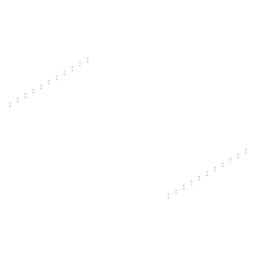
Shelf Support drillings for entire panel (Autodesk Fusion 360 design; units mm, degrees)
Autodesk Fusion 360 part; units mm, degrees
sketch "Control" plane through (0, 0, 0) normal (0, 0, 1) x (1, 0, 0)
  line L0 (378.5, -280) -> (-378.5, -280)
  line L1 (-378.5, -280) -> (-378.5, 280)
  line L2 (-378.5, 280) -> (378.5, 280)
  line L3 (378.5, 280) -> (378.5, -280)
  line L4 (378.5, -280) -> (-378.5, 280) construction
  line L5 (-378.5, -280) -> (378.5, 280) construction
  point P0 (0, 160)
  dimension "d7" = 560
  dimension "d8" = 757
  dimension "d9" = 378.5
  dimension "d100" = 120
  constraint horizontal L0
  constraint perpendicular L0 L1
  constraint parallel L0 L2
  constraint parallel L1 L3
  constraint coincident L4 origin
  constraint coincident L5 origin
  measures "d7" distance of L0.end L1.end
  measures "d8" distance of L1 L3
  measures "d9" distance of L1 P0
  measures "d100" vertical distance of L1.end P0
ref_plane "WorkPlane1" through (0, 160, 0) normal (0, 1, 0) x (0, 0, 1)
ref_plane "WorkPlane2" through (0, 0, 0) normal (1, 0, 0) x (0, 1, 0)
sketch "Sketch5" plane through (0, 0, 0) normal (0, 0, 1) x (1, 0, 0)
  line L0 (346.5, 160) -> (-346.5, 160) construction
  line L1 (-378.5, 280) -> (378.5, 280) construction
  line L2 (378.5, 280) -> (378.5, -280) construction
  line L3 (-378.5, -280) -> (-378.5, 280) construction
  circle A0 centre (-346.5, 160) radius 2.5
  circle A1 centre (346.5, 160) radius 2.5
  dimension "d116" = 120
  dimension "d117" = 32
  dimension "d118" = 32
  dimension "d119" = 5
  dimension "d120" = 5
  constraint horizontal L0
  constraint coincident L0.end A0.centre
  constraint coincident L0.start A1.centre
  measures "d116" distance of L0 L1
  measures "d117" distance of L0.end L3
  measures "d118" distance of L0.start L2
  measures "d119" diameter of A0
  measures "d120" diameter of A1
extrude "Extrude1" add sketch "Sketch5" along normal blind -12 and the other way blind -0.1 makes body 1 at (-346.9341, 162.462, -7.9667) makes body 2 at (346.0659, 162.462, -7.9667)
copy_body "Body->Comp1" bodies 1 removing the originals makes body 3 in component "Component"
copy_body "Body->Comp2" bodies 2 removing the originals makes body 4 in component "Component'"
pattern_linear "00000000-0000-0000-0000-000000000000" [suppressed]
component "Component" placed x (1, 0, 0) y (0, 1, 0) z (0, 0, 1) at (0, 0, 0)
component "Component'" placed x (1, 0, 0) y (0, 1, 0) z (0, 0, 1) at (0, 0, 0)
component "Component" placed x (1, 0, 0) y (0, 1, 0) z (0, 0, 1) at (0, -34, 0)
component "Component'" placed x (1, 0, 0) y (0, 1, 0) z (0, 0, 1) at (0, -34, 0)
component "Component" placed x (1, 0, 0) y (0, 1, 0) z (0, 0, 1) at (0, -68, 0)
component "Component'" placed x (1, 0, 0) y (0, 1, 0) z (0, 0, 1) at (0, -68, 0)
component "Component" placed x (1, 0, 0) y (0, 1, 0) z (0, 0, 1) at (0, -102, 0)
component "Component'" placed x (1, 0, 0) y (0, 1, 0) z (0, 0, 1) at (0, -102, 0)
component "Component" placed x (1, 0, 0) y (0, 1, 0) z (0, 0, 1) at (0, -136, 0)
component "Component'" placed x (1, 0, 0) y (0, 1, 0) z (0, 0, 1) at (0, -136, 0)
component "Component" placed x (1, 0, 0) y (0, 1, 0) z (0, 0, 1) at (0, -170, 0)
component "Component'" placed x (1, 0, 0) y (0, 1, 0) z (0, 0, 1) at (0, -170, 0)
component "Component" placed x (1, 0, 0) y (0, 1, 0) z (0, 0, 1) at (0, -204, 0)
component "Component'" placed x (1, 0, 0) y (0, 1, 0) z (0, 0, 1) at (0, -204, 0)
component "Component" placed x (1, 0, 0) y (0, 1, 0) z (0, 0, 1) at (0, -238, 0)
component "Component'" placed x (1, 0, 0) y (0, 1, 0) z (0, 0, 1) at (0, -238, 0)
component "Component" placed x (1, 0, 0) y (0, 1, 0) z (0, 0, 1) at (0, -272, 0)
component "Component'" placed x (1, 0, 0) y (0, 1, 0) z (0, 0, 1) at (0, -272, 0)
component "Component" placed x (1, 0, 0) y (0, 1, 0) z (0, 0, 1) at (0, -306, 0)
component "Component'" placed x (1, 0, 0) y (0, 1, 0) z (0, 0, 1) at (0, -306, 0)
component "Component" placed x (1, 0, 0) y (0, 1, 0) z (0, 0, 1) at (0, -340, 0)
component "Component'" placed x (1, 0, 0) y (0, 1, 0) z (0, 0, 1) at (0, -340, 0)
equation "FacadeWidth = 757.00 mm"
equation "FacadeHeight = 560.00 mm"
equation "HandleHorPos = FacadeWidth / 2"
equation "TopDistance = 120 mm"
equation "d7 = FacadeHeight"
equation "d8 = FacadeWidth"
equation "d9 = HandleHorPos"
equation "FacadeThickness = 18 mm"
equation "d100 = TopDistance"
equation "BottomDistance = 100 mm"
equation "FrontDistance = 32 mm"
equation "d116 = TopDistance"
equation "d117 = FrontDistance"
equation "d118 = d117"
equation "Spacing = 32 mm"
equation "Nbr_pin = floor(( FacadeHeight - TopDistance - BottomDistance ) / Spacing)"
equation "d131 = Nbr_pin + 1"
equation "d133 = ( -FacadeHeight + TopDistance + BottomDistance ) / Nbr_pin"
